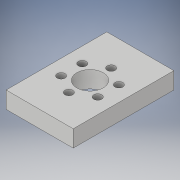
# Autodesk Inventor part: rev holes
Saved by Autodesk Inventor 2019 (Build 230136000, 136)
## iProperties
Created: 2019-11-03
Part Number: rev holes
Material: Generic
Document SubType Name: Modeling
Designer: shrey
Density: 1 g/cm^3
Appearance: Default
Author: shrey
Autodesk Inventor part; units mm, degrees
ref_plane "YZ Plane" through (0, 0, 0) normal (1, 0, 0) x (0, 1, 0)
ref_plane "XZ Plane" through (0, 0, 0) normal (0, 1, 0) x (-1, 0, 0)
ref_plane "XY Plane" through (0, 0, 0) normal (0, 0, 1) x (1, 0, 0)
sketch "Sketch1" plane through (0, 0, 0) normal (0, 1, 0) x (-1, 0, 0)
  circle A0 centre (0, 0) radius 8 construction
  circle A1 centre (0, -8) radius 1.5
  circle A2 centre (6.9282, -4) radius 1.5
  circle A3 centre (6.9282, 4) radius 1.5
  circle A4 centre (0, 8) radius 1.5
  circle A5 centre (-6.9282, 4) radius 1.5
  circle A6 centre (-6.9282, -4) radius 1.5
  circle A7 centre (0, 0) radius 5
  line L0 (12.7, 19.05) -> (-12.7, 19.05)
  line L1 (-12.7, 19.05) -> (-12.7, -19.05)
  line L2 (-12.7, -19.05) -> (12.7, -19.05)
  line L3 (12.7, -19.05) -> (12.7, 19.05)
  line L4 (12.7, 19.05) -> (-12.7, -19.05) construction
  line L5 (-12.7, 19.05) -> (12.7, -19.05) construction
  dimension "d0" = 16
  dimension "d1" = 3
  dimension "d4" = 360
  dimension "d6" = 10
  dimension "d7" = 25.4
  dimension "d8" = 38.1
  constraints: 12 end point, 7 centre point, 2 coincident, 2 midpoint, 2 parallel, 1 horizontal, 1 perpendicular, 1 vertical alignment, 15 other
  measures "d1" diameter of A1
  measures "d6" diameter of A7
  measures "d7" distance of L2.end L1.end
  measures "d8" distance of L0.end L1.end
extrude "Extrusion1" add sketch "Sketch1" along normal blind 6.35
body "Solid1"
